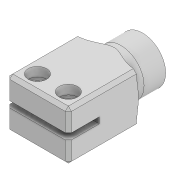
# Autodesk Inventor part: Holder
Saved by Autodesk Inventor 2020 (Build 240168000, 168)
## iProperties
Created: 2021-10-15
Part Number: Holder
Material: Generic
Document SubType Name: Modeling
Designer: ferrerx
Density: 1 g/cm^3
Appearance: Default
Author: ferrerx
Autodesk Inventor part; units mm, degrees
ref_plane "YZ Plane" through (0, 0, 0) normal (1, 0, 0) x (0, 1, 0)
ref_plane "XZ Plane" through (0, 0, 0) normal (0, 1, 0) x (-1, 0, 0)
ref_plane "XY Plane" through (0, 0, 0) normal (0, 0, 1) x (1, 0, 0)
sketch "Sketch1" plane through (0, 0, 0) normal (0, 1, 0) x (-1, 0, 0)
  line L0 (-10, -5) -> (10, -5)
  line L1 (10, -5) -> (10, 5)
  line L2 (10, 5) -> (-10, 5)
  line L3 (-10, 5) -> (-10, -5)
  line L4 (-10, -5) -> (10, 5) construction
  line L5 (10, -5) -> (-10, 5) construction
  circle A0 centre (5, 0) radius 1.55
  circle A1 centre (-5, 0) radius 1.55
  line L6 (10, -5) -> (-10, -5)
  line L7 (-10, -5) -> (-10, -17)
  line L8 (-10, -17) -> (10, -17)
  line L9 (10, -17) -> (10, -5)
  point P0 (0, 0)
  dimension "d0" = 3.1
  dimension "d1" = 3.1
  dimension "d2" = 20
  dimension "d3" = 10
  dimension "d4" = 5
  dimension "d5" = 10
  dimension "d8" = 12
  constraints: 20 end point, 4 parallel, 2 centre point, 2 horizontal, 2 midpoint, 2 perpendicular
  measures "d0" diameter of A0
  measures "d1" diameter of A1
  measures "d2" distance of L0.start L0.end
  measures "d3" distance of A0.centre A1.centre
  measures "d4" distance of point (0, 0) A1.centre
  measures "d5" distance of L0.end L1.end
  measures "d8" distance of L6.end L7.end
extrude "Extrusion1" add sketch "Sketch1" along normal blind 16
sketch "Sketch2" plane through (10, 0, 5) normal (1, 0, 0) x (0, 0, -1)
  line L0 (0, 0) -> (0, 16) projected
  line L1 (0, 8) -> (4.5, 8)
  line L2 (10, 9) -> (-1, 9)
  line L3 (-1, 9) -> (-1, 7)
  line L4 (-1, 7) -> (10, 7)
  line L5 (10, 7) -> (10, 9)
  line L6 (10, 9) -> (-1, 7) construction
  line L7 (-1, 9) -> (10, 7) construction
  line L8 (0, 16) -> (22, 16) projected
  point P0 (5, 0)
  point P1 (0, 9)
  point P2 (0, 7)
  dimension "d9" = 11
  dimension "d13" = 2
  dimension "d14" = 4.5
  constraints: 14 end point, 3 midpoint, 2 parallel, 1 horizontal, 1 perpendicular
  measures "d9" distance of L3.end L4.end
  measures "d13" distance of L2.end L3.end
  measures "d14" distance of L1.start L1.end
extrude "Extrusion2" cut sketch "Sketch2" against normal blind 24.75 contours L0 L2 L5 L4
sketch "Sketch3" plane through (10, 0, -17) normal (0, 0, -1) x (-1, 0, 0)
  line L0 (10, 0) -> (10, 16) construction
  circle A0 centre (10, 8) radius 7.5
  line L1 (0, 16) -> (20, 16) projected
  dimension "d15" = 15
  constraints: 2 end point, 2 midpoint, 1 centre point
  measures "d15" diameter of A0
extrude "Extrusion3" add sketch "Sketch3" along normal blind 12 and the other way blind 12
sketch "Sketch4" plane through (0, 8, -29) normal (0, 0, -1) x (-1, 0, 0)
  circle A0 centre (0, 0) radius 5
  point P0 (0, -8)
  dimension "d20" = 10
  constraints: 1 centre point
  measures "d20" diameter of A0
extrude "Extrusion4" cut sketch "Sketch4" against normal blind 14
sketch "Sketch5" plane through (0, 16, 0) normal (0, 1, 0) x (1, 0, 0)
  circle A0 centre (5, 0) radius 1.55 projected
  circle A1 centre (5, 0) radius 3
  circle A2 centre (-5, 0) radius 1.55 projected
  circle A3 centre (-5, 0) radius 3
  point P0 (0, 0)
  dimension "d23" = 6
  dimension "d24" = 6
  constraints: 2 centre point, 2 coincident
  measures "d23" diameter of A1
  measures "d24" diameter of A3
extrude "Extrusion5" cut sketch "Sketch5" against normal blind 3 contours A0 | A1 | A2 | A3
sketch "Sketch6" plane through (0, 0, 0) normal (0, -1, 0) x (1, 0, 0)
  circle A0 centre (5, 0) radius 1.55 projected
  line L0 (8.4641, 0) -> (6.7321, -3)
  line L1 (6.7321, -3) -> (3.2679, -3)
  line L2 (3.2679, -3) -> (1.5359, 0)
  line L3 (1.5359, 0) -> (3.2679, 3)
  line L4 (3.2679, 3) -> (6.7321, 3)
  line L5 (6.7321, 3) -> (8.4641, 0)
  circle A1 centre (-5, 0) radius 1.55 projected
  line L6 (-1.5359, 0) -> (-3.2679, -3)
  line L7 (-3.2679, -3) -> (-6.7321, -3)
  line L8 (-6.7321, -3) -> (-8.4641, 0)
  line L9 (-8.4641, 0) -> (-6.7321, 3)
  line L10 (-6.7321, 3) -> (-3.2679, 3)
  line L11 (-3.2679, 3) -> (-1.5359, 0)
  line L12 (-10, 5) -> (10, 5) projected
  point P0 (0, 0)
  dimension "d27" = 6
  dimension "d28" = 6
  constraints: 24 end point, 2 coincident, 2 parallel, 26 other
  measures "d27" distance between parallel lines of L1 L4
  measures "d28" distance between parallel lines of L10 L7
extrude "Extrusion6" cut sketch "Sketch6" against normal blind 3
fillet "Fillet1" radius 5 1 edges at (7.5, 8, -17)
chamfer "Chamfer1" distance 1 angle 45 10 edges at (-10, 16, -6) (10, 16, -6) (0, 16, 5) (10, 12.5, 5) (-10, 12.5, 5) (-10, 3.5, 5) (10, 3.5, 5) (0, 0, 5) (10, 0, -6) (-10, 0, -6)
body "Solid1"
